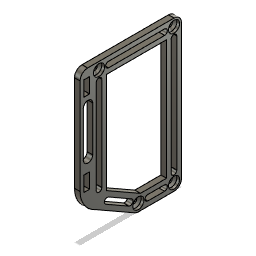
sidemount_b (Autodesk Fusion 360 design; units mm, degrees)
Autodesk Fusion 360 part; units mm, degrees
sketch "Sketch1" plane through (0, 0, 0) normal (1, 0, 0) x (0, 0, -1)
  circle A0 centre (0, 0) radius 1.5
  line L0 (0, 0) -> (19, 0)
  line L1 (19, 0) -> (19, 72)
  line L2 (19, 72) -> (-21, 72)
  circle A1 centre (19, 0) radius 1.5
  circle A2 centre (19, 72) radius 1.5
  circle A3 centre (-21, 72) radius 1.5
  circle A4 centre (0, 0) radius 4
  circle A5 centre (19, 0) radius 4
  circle A6 centre (19, 72) radius 4
  circle A7 centre (-21, 72) radius 4
  line L3 (-21, 72) -> (-21, 12)
  line L4 (-21, 12) -> (0, 0)
  circle A8 centre (-21, 12) radius 4
  line L5 (-21, 12) -> (-22.9846, 8.527)
  line L6 (-22.9846, 8.527) -> (-1.9846, -3.473)
  line L7 (-21, 12) -> (-19.0154, 15.473)
  line L8 (-19.0154, 15.473) -> (1.9846, 3.473)
  line L9 (0, -4) -> (19, -4)
  line L10 (19, 4) -> (0, 4)
  line L11 (15, 0) -> (15, 72)
  line L12 (23, 0) -> (23, 72)
  line L13 (19, 76) -> (-21, 76)
  line L14 (-21, 68) -> (19, 68)
  line L15 (-17, 72) -> (-17, 12)
  line L16 (-21, 76) -> (-24.2353, 76)
  line L17 (-24.2353, 72) -> (-24.2353, 76)
  line L18 (15, 68) -> (15, 71.012)
  line L19 (-17, 68) -> (-17, 70)
  line L20 (-17, 14.3213) -> (-17, 11.7242)
  line L21 (-31.0898, 70.9307) -> (-31.0898, 20.9307)
  arc A9 (-31.0898, 20.9307) -> (-22.9846, 8.527) centre (-17.5463, 20.9307) ccw
  line L22 (-27.0898, 76) -> (-27.0898, 72)
  arc A10 (-27.0898, 76) -> (-31.0898, 72) centre (-27.0898, 72) ccw
  line L23 (-24.2353, 76) -> (-27.0898, 76)
  line L24 (-31.0898, 72) -> (-31.0898, 70.9307)
  dimension "d1" = 3
  dimension "d2" = 19
  dimension "d3" = 72
  dimension "d4" = 40
  dimension "d5" = 3
  dimension "d6" = 3
  dimension "d7" = 3
  dimension "d8" = 8
  dimension "d9" = 8
  dimension "d10" = 8
  dimension "d11" = 8
  dimension "d12" = 60
  dimension "d13" = 8
  dimension "d34" = 2
  dimension "d81" = 50
  dimension "d124" = 4
  constraint coincident A0.centre L0.start
  constraint horizontal L0
  constraint perpendicular L0 L1
  constraint perpendicular L1 L2
  constraint coincident L0.end L1.start
  constraint coincident L1.end L2.start
  constraint coincident L2.end A3.centre
  constraint concentric A0 A4
  constraint concentric A1 A5
  constraint concentric A2 A6
  constraint concentric A3 A7
  constraint perpendicular L2 L3
  constraint coincident L3.end L4.start
  constraint coincident A8 L5.end
  constraint perpendicular L4 L5
  constraint coincident A4 L6.end
  constraint tangent A4 L6
  constraint coincident A8 L7.end
  constraint perpendicular L6 L7
  constraint coincident A4 L8.end
  constraint tangent A4 L8
  constraint coincident A4 L9.start
  constraint coincident A5 L9.end
  constraint tangent A5 L9
  constraint horizontal L9
  constraint coincident A5 L10.start
  constraint coincident L1 L10.start
  constraint coincident A4 L10.end
  constraint tangent A4 L10
  constraint coincident A5 L11.start
  constraint coincident L0 L11.start
  constraint coincident A6 L11.end
  constraint coincident L2 L11.end
  constraint coincident A5 L12.start
  constraint coincident A6 L12.end
  constraint tangent A6 L12
  constraint parallel L11 L12
  constraint coincident A6 L13.start
  constraint coincident A7 L13.end
  constraint tangent A7 L13
  constraint perpendicular L12 L13
  constraint coincident A7 L14.start
  constraint coincident L3 L14.start
  constraint coincident A6 L14.end
  constraint coincident L1 L14.end
  constraint coincident A7 L15.start
  constraint coincident L2 L15.start
  constraint coincident A8 L15.end
  constraint tangent A8 L15
  constraint tangent A7 L16
  constraint vertical L17
  constraint coincident L14 L18.start
  constraint coincident L11 L18.start
  constraint perpendicular L14 L18
  constraint coincident L14 L19.start
  constraint coincident L15 L19.start
  constraint perpendicular L14 L19
  constraint coincident L8 L20.start
  constraint coincident L15 L20.start
  constraint parallel L15 L20
  constraint vertical L21
  constraint tangent L21 A9
  constraint coincident L22.end A10.centre
  constraint tangent A10 L23
  constraint tangent A10 L24
  measures "d1" diameter of A0
  measures "d2" distance of A0.centre L0.end
  measures "d3" distance of L0.end L1.end
  measures "d4" distance of L1.end L2.end
  measures "d5" diameter of A1
  measures "d6" diameter of A2
  measures "d7" diameter of A3
  measures "d8" diameter of A4
  measures "d9" diameter of A5
  measures "d10" diameter of A6
  measures "d11" diameter of A7
  measures "d12" distance of L2.end L3.end
  measures "d13" diameter of A8
  measures "d34" distance of L19.start L19.end
  measures "d81" distance of L21.start L21.end
  measures "d124" distance of L22.start L22.end
extrude "Extrude1" add sketch "Sketch1" along normal blind 3 contours A0 L0 A4 L4 | A0 L0 A4 L4 | L0 A4 L8 L10 L11 | L0 A4 A5 L9 | A4 L4 A8 L8 L10 L15 L20 | A4 L4 A8 L6 | L0 L1 A1 A5 | A5 L10 L11 | L0 L1 A1 A5 | A4 L8 L10 | L4 A8 L5 | L4 A8 L7 | L1 L10 L11 L14 | L1 A5 A6 L12 | A7 L3 A8 L17 L21 A9 A10 L23 L24 | L3 A8 L5 | L3 A8 L7 | A8 L8 L15 L20 | L1 L2 A2 A6 | A6 L11 L14 L18 | L1 L2 A2 A6 | L2 L11 L14 L15 L18 L19 | L3 A8 L8 L14 L15 | L2 A6 A7 L13 | A7 L14 L15 L19 | L2 A3 A7 L3 | L2 A3 A7 L3 | A7 L16 L17
sketch "Sketch2" plane through (0, 0, 0) normal (-1, 0, 0) x (0, 0, 1)
  circle A0 centre (21, 72) radius 1.5
  circle A1 centre (0, 0) radius 1.5
  circle A2 centre (-19, 0) radius 1.5
  circle A3 centre (-19, 72) radius 1.5
  line L0 (27.0898, 76) -> (-19, 76)
  arc A4 (-19, 76) -> (-23, 72) centre (-19, 72) ccw
  line L1 (-23, 72) -> (-23, 0)
  arc A5 (-23, 0) -> (-19, -4) centre (-19, 0) ccw
  line L2 (-19, -4) -> (0, -4)
  arc A6 (0, -4) -> (1.9846, -3.473) centre (0, 0) ccw
  line L3 (1.9846, -3.473) -> (22.9846, 8.527)
  line L4 (17, 14.3213) -> (-1.0623, 4)
  line L5 (-1.0623, 4) -> (-15, 4)
  line L6 (-15, 4) -> (-15, 68)
  line L7 (-15, 68) -> (17, 68)
  line L8 (17, 68) -> (17, 14.3213)
  line L9 (27.958, 63.4995) -> (27.958, 71.4995)
  arc A7 (22.9846, 8.527) -> (31.0898, 20.9307) centre (17.5463, 20.9307) ccw
  line L10 (31.0898, 20.9307) -> (31.0898, 72)
  line L11 (31.0898, 27.4995) -> (29.0898, 27.4995)
  line L12 (31.0898, 63.4995) -> (29.0898, 63.4995)
  line L13 (29.0898, 63.4995) -> (26.0898, 63.4995)
  line L14 (26.0898, 63.4995) -> (26.0898, 71.4995)
  line L15 (26.0898, 71.4995) -> (29.0898, 71.4995)
  line L16 (29.0898, 71.4995) -> (29.0898, 63.4995)
  line L17 (29.0898, 27.4995) -> (26.0898, 27.4995)
  line L18 (26.0898, 27.4995) -> (26.0898, 19.4995)
  line L19 (26.0898, 19.4995) -> (29.0898, 19.4995)
  line L20 (29.0898, 19.4995) -> (29.0898, 27.4995)
  arc A8 (31.0898, 72) -> (27.0898, 76) centre (27.0898, 72) ccw
  dimension "d78" = 8
  dimension "d110" = 2
  dimension "d111" = 2
  dimension "d112" = 3
  dimension "d113" = 3
  dimension "d114" = 8
  constraint vertical L9
  constraint coincident L10 L11.start
  constraint perpendicular L10 L11
  constraint coincident L10 L12.start
  constraint perpendicular L10 L12
  constraint horizontal L13
  constraint vertical L14
  constraint horizontal L15
  constraint vertical L16
  constraint horizontal L17
  constraint vertical L18
  constraint horizontal L19
  constraint vertical L20
  measures "d78" distance of L9.end L9.start
  measures "d110" distance of L11.start L11.end
  measures "d111" distance of L12.start L12.end
  measures "d112" distance of L12.end L13.end
  measures "d113" distance of L11.end L17.end
  measures "d114" distance of L11.end L19.end
extrude "Extrude2" cut sketch "Sketch2" against normal blind 3 contours L9 L13 L14 L15 | L9 L13 L15 L16 | L17 L18 L19 L20
sketch "Sketch3" plane through (0, 0, 0) normal (-1, 0, 0) x (0, 0, 1)
  circle A0 centre (-19, 72) radius 1.5
  circle A1 centre (-19, 0) radius 1.5
  circle A2 centre (0, 0) radius 1.5
  circle A3 centre (21, 72) radius 1.5
  line L0 (17, 14.3213) -> (-1.0623, 4)
  line L1 (-1.0623, 4) -> (-15, 4)
  line L2 (-15, 4) -> (-15, 68)
  line L3 (-15, 68) -> (17, 68)
  line L4 (17, 68) -> (17, 14.3213)
  line L5 (27.0898, 76) -> (-19, 76)
  arc A4 (-19, 76) -> (-23, 72) centre (-19, 72) ccw
  line L6 (-23, 72) -> (-23, 0)
  arc A5 (-23, 0) -> (-19, -4) centre (-19, 0) ccw
  line L7 (-19, -4) -> (0, -4)
  arc A6 (0, -4) -> (1.9846, -3.473) centre (0, 0) ccw
  line L8 (1.9846, -3.473) -> (22.9846, 8.527)
  line L9 (-19, 72) -> (-19, 0)
  line L10 (-19, 0) -> (0, 0)
  line L11 (0, 0) -> (21, 12)
  line L12 (21, 72) -> (-19, 72)
  line L13 (-19, 72) -> (-19, 67)
  line L14 (-19, 0) -> (-19, 5)
  circle A7 centre (-19, 5) radius 1.5
  circle A8 centre (-19, 67) radius 1.5
  line L15 (-17.5, 67) -> (-17.5, 5)
  line L16 (-20.5, 5) -> (-20.5, 67)
  line L17 (-19, 0) -> (-14, 0)
  line L18 (0, 0) -> (-5, 0)
  line L19 (0, 0) -> (4.3412, 2.4807)
  line L20 (21, 12) -> (16.6588, 9.5193)
  line L21 (21, 72) -> (16, 72)
  line L22 (-19, 72) -> (-14, 72)
  circle A9 centre (-14, 72) radius 1.5
  circle A10 centre (16, 72) radius 1.5
  circle A11 centre (16.6588, 9.5193) radius 1.5
  circle A12 centre (4.3412, 2.4807) radius 1.5
  circle A13 centre (-5, 0) radius 1.5
  circle A14 centre (-14, 0) radius 1.5
  line L23 (-14, -1.5) -> (-5, -1.5)
  line L24 (-5, 1.5) -> (-14, 1.5)
  line L25 (16.6588, 9.5193) -> (17.403, 8.2169)
  line L26 (17.403, 8.2169) -> (5.0854, 1.1783)
  line L27 (16.6588, 9.5193) -> (15.9146, 10.8217)
  line L28 (15.9146, 10.8217) -> (3.597, 3.7831)
  line L29 (16, 70.5) -> (-14, 70.5)
  line L30 (-14, 73.5) -> (16, 73.5)
  line L31 (21, 72) -> (20, 72)
  arc A15 (22.9846, 8.527) -> (31.0898, 20.9307) centre (17.5463, 20.9307) ccw
  line L32 (31.0898, 20.9307) -> (31.0898, 72)
  line L33 (21, 12) -> (21, 17)
  line L34 (21, 72) -> (21, 67)
  circle A16 centre (21, 67) radius 1.5
  circle A17 centre (21, 17) radius 1.5
  line L35 (22.5, 17) -> (22.5, 67)
  line L36 (19.5, 67) -> (19.5, 17)
  line L37 (29.0898, 71.4995) -> (29.0898, 63.4995)
  line L38 (29.0898, 63.4995) -> (26.0898, 63.4995)
  line L39 (26.0898, 63.4995) -> (26.0898, 71.4995)
  line L40 (26.0898, 71.4995) -> (29.0898, 71.4995)
  line L41 (26.0898, 27.4995) -> (29.0898, 27.4995)
  line L42 (29.0898, 27.4995) -> (29.0898, 19.4995)
  line L43 (29.0898, 19.4995) -> (26.0898, 19.4995)
  line L44 (26.0898, 19.4995) -> (26.0898, 27.4995)
  arc A18 (31.0898, 72) -> (27.0898, 76) centre (27.0898, 72) ccw
  dimension "d38" = 5
  dimension "d39" = 5
  dimension "d40" = 3
  dimension "d41" = 3
  dimension "d42" = 5
  dimension "d43" = 5
  dimension "d44" = 5
  dimension "d45" = 5
  dimension "d48" = 5
  dimension "d49" = 5
  dimension "d50" = 3
  dimension "d51" = 3
  dimension "d54" = 3
  dimension "d55" = 3
  dimension "d56" = 3
  dimension "d57" = 3
  dimension "d66" = 1
  dimension "d82" = 5
  dimension "d83" = 5
  dimension "d84" = 3
  dimension "d85" = 3
  constraint coincident A0.centre A4.centre
  constraint coincident A1.centre A5.centre
  constraint coincident A2.centre A6.centre
  constraint coincident A3.centre L12.start
  constraint perpendicular L12 L13
  constraint perpendicular L10 L14
  constraint coincident L14.end A7.centre
  constraint coincident L13.end A8.centre
  constraint coincident A8 L15.start
  constraint coincident A7 L15.end
  constraint tangent A7 L15
  constraint perpendicular L10 L15
  constraint coincident A7 L16.start
  constraint coincident A8 L16.end
  constraint tangent A8 L16
  constraint perpendicular L5 L16
  constraint perpendicular L14 L17
  constraint parallel L10 L18
  constraint parallel L11 L19
  constraint parallel L11 L20
  constraint perpendicular L9 L22
  constraint coincident L22.end A9.centre
  constraint coincident L21.end A10.centre
  constraint coincident L20.end A11.centre
  constraint coincident L19.end A12.centre
  constraint coincident L18.end A13.centre
  constraint coincident L17.end A14.centre
  constraint coincident A14 L23.start
  constraint coincident A13 L23.end
  constraint tangent A13 L23
  constraint horizontal L23
  constraint coincident A13 L24.start
  constraint coincident A14 L24.end
  constraint tangent A14 L24
  constraint parallel L18 L24
  constraint coincident A11 L25.end
  constraint perpendicular L11 L25
  constraint coincident A12 L26.end
  constraint tangent A12 L26
  constraint coincident A11 L27.end
  constraint perpendicular L11 L27
  constraint coincident A12 L28.end
  constraint tangent A12 L28
  constraint coincident A10 L29.start
  constraint coincident A9 L29.end
  constraint tangent A9 L29
  constraint perpendicular L13 L29
  constraint coincident A9 L30.start
  constraint coincident A10 L30.end
  constraint tangent A10 L30
  constraint perpendicular L13 L30
  constraint vertical L33
  constraint perpendicular L21 L34
  constraint coincident L34.end A16.centre
  constraint coincident L33.end A17.centre
  constraint coincident A17 L35.start
  constraint coincident A16 L35.end
  constraint tangent A16 L35
  constraint vertical L35
  constraint coincident A16 L36.start
  constraint coincident A17 L36.end
  constraint tangent A17 L36
  constraint parallel L33 L36
  measures "d38" distance of A0.centre L13.end
  measures "d39" distance of A1.centre L14.end
  measures "d40" diameter of A7
  measures "d41" diameter of A8
  measures "d42" distance of A1.centre L17.end
  measures "d43" distance of A2.centre L18.end
  measures "d44" distance of A2.centre L19.end
  measures "d45" distance of L11.end L20.end
  measures "d48" distance of A3.centre L21.end
  measures "d49" distance of A0.centre L22.end
  measures "d50" diameter of A9
  measures "d51" diameter of A10
  measures "d54" diameter of A11
  measures "d55" diameter of A12
  measures "d56" diameter of A13
  measures "d57" diameter of A14
  measures "d66" distance of A3.centre L31.end
  measures "d82" distance of L11.end L33.end
  measures "d83" distance of A3.centre L34.end
  measures "d84" diameter of A16
  measures "d85" diameter of A17
extrude "Extrude3" cut sketch "Sketch3" against normal blind 3 contours L12 L22 A9 | L12 L22 A9 | L9 L13 A8 | L9 L13 A8 | L12 A9 A10 L30 | L12 A9 A10 L29 | L9 A7 A8 L15 | L9 A7 A8 L16 | L12 L21 A10 | L12 L21 A10 | L9 L14 A7 | L9 L14 A7 | A16 | L10 L17 A14 | L10 L17 A14 | A16 A17 L35 L36 | L10 A13 A14 L24 | L10 A13 A14 L23 | A17 | L10 L18 A13 | L10 L18 A13 | L11 L20 A11 L25 | L11 L20 A11 L27 | L11 A11 L25 | L11 A11 L27 | L11 A11 A12 L28 | L11 L19 A12 | L11 L19 A12 | L11 A11 A12 L26
hole "Hole5" at (3, 72, 21) direction (-1, 0, 0) diameter 6 depth 1.5 tip angle 118
hole "Hole6" at (3, 72, -19) direction (-1, 0, 0) diameter 6 depth 1.5 tip angle 118
hole "Hole7" at (3, 0, -19) direction (-1, 0, 0) diameter 6 depth 1.5 tip angle 118
hole "Hole8" at (3, 0, 0) direction (-1, 0, 0) diameter 6 depth 1.5 tip angle 118
sketch "Sketch5" plane through (3, 0, 0) normal (1, 0, 0) x (0, 0, -1)
  circle A0 centre (0, 0) radius 3
  circle A1 centre (19, 0) radius 3
  circle A2 centre (19, 72) radius 3
  circle A3 centre (-21, 72) radius 3
  arc A4 (14, -1.5) -> (14, 1.5) centre (14, 0) ccw
  line L0 (14, -1.5) -> (5, -1.5)
  arc A5 (5, 1.5) -> (5, -1.5) centre (5, 0) ccw
  line L1 (5, 1.5) -> (14, 1.5)
  line L2 (-15.9146, 10.8217) -> (-3.597, 3.7831)
  arc A6 (-5.0854, 1.1783) -> (-3.597, 3.7831) centre (-4.3412, 2.4807) ccw
  line L3 (-5.0854, 1.1783) -> (-17.403, 8.2169)
  arc A7 (-15.9146, 10.8217) -> (-17.403, 8.2169) centre (-16.6588, 9.5193) ccw
  line L4 (20.5, 67) -> (20.5, 5)
  arc A8 (17.5, 5) -> (20.5, 5) centre (19, 5) ccw
  line L5 (17.5, 5) -> (17.5, 67)
  arc A9 (20.5, 67) -> (17.5, 67) centre (19, 67) ccw
  line L6 (14, 70.5) -> (-16, 70.5)
  arc A10 (-16, 73.5) -> (-16, 70.5) centre (-16, 72) ccw
  line L7 (-16, 73.5) -> (14, 73.5)
  arc A11 (14, 70.5) -> (14, 73.5) centre (14, 72) ccw
  arc A12 (-22.5, 17) -> (-19.5, 17) centre (-21, 17) ccw
  line L8 (-22.5, 17) -> (-22.5, 67)
  arc A13 (-19.5, 67) -> (-22.5, 67) centre (-21, 67) ccw
  line L9 (-19.5, 67) -> (-19.5, 17)
  line L10 (-26.0898, 71.4995) -> (-26.0898, 63.4995)
  line L11 (-26.0898, 63.4995) -> (-29.0898, 63.4995)
  line L12 (-29.0898, 63.4995) -> (-29.0898, 71.4995)
  line L13 (-29.0898, 71.4995) -> (-26.0898, 71.4995)
  line L14 (-29.0898, 27.4995) -> (-26.0898, 27.4995)
  line L15 (-26.0898, 27.4995) -> (-26.0898, 19.4995)
  line L16 (-26.0898, 19.4995) -> (-29.0898, 19.4995)
  line L17 (-29.0898, 19.4995) -> (-29.0898, 27.4995)
  line L18 (-17, 68) -> (15, 68)
  line L19 (15, 68) -> (15, 4)
  line L20 (15, 4) -> (1.0623, 4)
  line L21 (1.0623, 4) -> (-17, 14.3213)
  line L22 (-17, 14.3213) -> (-17, 68)
  line L23 (19, 76) -> (-27.0898, 76)
  line L24 (-31.0898, 72) -> (-31.0898, 20.9307)
  arc A14 (-31.0898, 20.9307) -> (-22.9846, 8.527) centre (-17.5463, 20.9307) ccw
  line L25 (-22.9846, 8.527) -> (-1.9846, -3.473)
  arc A15 (-1.9846, -3.473) -> (0, -4) centre (0, 0) ccw
  line L26 (0, -4) -> (19, -4)
  arc A16 (19, -4) -> (23, 0) centre (19, 0) ccw
  line L27 (23, 0) -> (23, 72)
  arc A17 (23, 72) -> (19, 76) centre (19, 72) ccw
  line L28 (-31.0898, 46.4653) -> (-26.8483, 46.4653)
  line L29 (-26.8483, 46.4653) -> (-26.8483, 58.4653)
  circle A18 centre (-26.8483, 58.4653) radius 2.5
  line L30 (-26.8483, 46.4653) -> (-26.8483, 34.4653)
  circle A19 centre (-26.8483, 34.4653) radius 2.5
  line L31 (-26.8483, 34.4653) -> (-24.3483, 34.4653)
  line L32 (-24.3483, 34.4653) -> (-24.3483, 46.4653)
  line L33 (-24.3483, 46.4653) -> (-24.3483, 58.4653)
  line L34 (-29.3483, 58.4653) -> (-29.3483, 34.4653)
  arc A20 (-27.0898, 76) -> (-31.0898, 72) centre (-27.0898, 72) ccw
  dimension "d115" = 4.2415
  dimension "d117" = 12
  dimension "d118" = 5
  dimension "d119" = 12
  dimension "d120" = 5
  constraint midpoint L24 L28.start
  constraint perpendicular L8 L28
  constraint perpendicular L28 L29
  constraint coincident L29.end A18.centre
  constraint perpendicular L28 L30
  constraint coincident L30.end A19.centre
  constraint coincident A19 L31.end
  constraint perpendicular L30 L31
  constraint coincident A18 L33.end
  constraint tangent A18 L33
  constraint coincident A18 L34.start
  constraint coincident A19 L34.end
  constraint tangent A19 L34
  constraint parallel L33 L34
  measures "d115" distance of L28.start L28.end
  measures "d117" distance of L28.end L29.end
  measures "d118" diameter of A18
  measures "d119" distance of L28.end L30.end
  measures "d120" diameter of A19
extrude "Extrude5" cut sketch "Sketch5" against normal blind 3 contours L28 L29 A18 L34 | L28 L30 A19 L34 | L29 A18 L30 A19 L32 L33 | A18 | L30 A19 L31 | L30 A19 L31
equation "d115 = 8.483 mm / 2"
